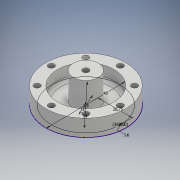
# Autodesk Inventor part: MoldeB
Saved by Autodesk Inventor 2017 (Build 210142000, 142)
## iProperties
Created: 2017-07-09
Part Number: MoldeB
Material: Generic
Document SubType Name: Modeling
Designer: LeoAlvarez
Density: 1 g/cm^3
Appearance: Default
Author: LeoAlvarez
Autodesk Inventor part; units mm, degrees
ref_plane "YZ Plane" through (0, 0, 0) normal (1, 0, 0) x (0, 1, 0)
ref_plane "XZ Plane" through (0, 0, 0) normal (0, 1, 0) x (-1, 0, 0)
ref_plane "XY Plane" through (0, 0, 0) normal (0, 0, 1) x (1, 0, 0)
sketch "Sketch1" plane through (0, 0, 0) normal (0, 0, 1) x (1, 0, 0)
  circle A0 centre (0, 0) radius 1.8
  circle A1 centre (0, 0) radius 17
  circle A2 centre (0, 0) radius 7.5
  circle A3 centre (0, 0) radius 24
  circle A4 centre (20.75, 0) radius 1.8
  circle A5 centre (14.6725, 14.6725) radius 1.8
  circle A6 centre (0, 20.75) radius 1.8
  circle A7 centre (-14.6725, 14.6725) radius 1.8
  circle A8 centre (-20.75, 0) radius 1.8
  circle A9 centre (-14.6725, -14.6725) radius 1.8
  circle A10 centre (0, -20.75) radius 1.8
  circle A11 centre (14.6725, -14.6725) radius 1.8
  dimension "d0" = 3.6
  dimension "d1" = 34
  dimension "d2" = 15
  dimension "d3" = 48
  dimension "d4" = 3.6
  dimension "d5" = 20.75
  dimension "d8" = 360
  constraints: 12 centre point, 4 coincident, 17 other
  measures "d0" diameter of A0
  measures "d1" diameter of A1
  measures "d2" diameter of A2
  measures "d3" diameter of A3
  measures "d4" diameter of A4
  measures "d5" distance of A4.centre point (0, 0)
extrude "Extrusion1" add sketch "Sketch1" along normal blind 2 contours A1 | A2 | A3
extrude "Extrusion2" add sketch "Sketch1" along normal blind 10 contours A3
fillet "Fillet1" radius 2 1 edges at (-17, 0, 2)
extrude "Extrusion3" add sketch "Sketch1" along normal blind 18 contours A2
body "Solid1"
